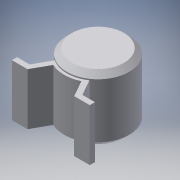
# Autodesk Inventor part: Motor
Saved by Autodesk Inventor 2019 (Build 230136000, 136)
## iProperties
Created: 2017-01-18
Part Number: Motor
Document SubType Name: Modeling
Designer: Administrator
Density: 1 g/cm^3
Mass: 12.288 g
Surface Area: 37.6061 cm^2
Volume: 12.288 cm^3
Material: Generic
Appearance: Cool White
Author: Administrator
Autodesk Inventor part; units mm, degrees
ref_plane "YZ Plane" through (0, 0, 0) normal (1, 0, 0) x (0, 1, 0)
ref_plane "XZ Plane" through (0, 0, 0) normal (0, 1, 0) x (-1, 0, 0)
ref_plane "XY Plane" through (0, 0, 0) normal (0, 0, 1) x (1, 0, 0)
sketch "Sketch1" plane through (0, 0, 0) normal (0, 0, 1) x (1, 0, 0)
  line L0 (0, 0) -> (0, -18.18) construction
  line L1 (0, -18.18) -> (-15, -18.18) construction
  line L2 (-15, -18.18) -> (-15, -16.18)
  line L3 (-15, -16.18) -> (-9, -16.18) construction
  line L4 (-9, -16.18) -> (0, 0) construction
  line L5 (-10.1443, -16.18) -> (-6.6868, -9.9643)
  line L6 (-5.4267, -11.8132) -> (-8.9682, -18.18)
  line L7 (-15, -16.18) -> (-10.1443, -16.18)
  line L8 (-15, -18.18) -> (-8.9682, -18.18)
  line L9 (15, -18.18) -> (15, -16.18)
  line L10 (15, -16.18) -> (9, -16.18) construction
  line L11 (10.1443, -16.18) -> (6.6868, -9.9643)
  line L12 (5.4267, -11.8132) -> (8.9682, -18.18)
  line L13 (15, -16.18) -> (10.1443, -16.18)
  line L14 (15, -18.18) -> (8.9682, -18.18)
  arc A0 (-5.4267, -11.8132) -> (5.4267, -11.8132) centre (0, 0) ccw
  arc A1 (6.6868, -9.9643) -> (-6.6868, -9.9643) centre (0, 0) ccw
  dimension "d1" = 15
  dimension "d2" = 18.18
  dimension "d3" = 2
  dimension "d4" = 6
  dimension "d5" = 1
  dimension "d6" = 2
  dimension "d9" = 12
  dimension "d10" = 13
  constraints: 30 end point, 7 symmetric about line, 4 parallel, 4 point on circle, 3 point on line, 2 centre point, 2 collinear, 1 perpendicular, 1 vertical, 1 other
  measures "d1" distance of L0.end L1.end
  measures "d2" distance from line of L0.start L1
  measures "d3" distance between parallel lines of L3 L1
  measures "d4" distance from line of L3.end L2
  measures "d5" distance between parallel lines of L5 L4
  measures "d6" distance between parallel lines of L5 L6
  measures "d9" radius of A1
  measures "d10" radius of A0
extrude "Extrusion1" add sketch "Sketch1" along normal mid plane 20
sketch "Sketch2" plane through (0, 0, 0) normal (0, 0, 1) x (1, 0, 0)
  arc A0 (6.6868, -9.9643) -> (-6.6868, -9.9643) centre (0, 0) ccw projected
  circle A1 centre (0, 0) radius 12
  constraints: 1 centre point, 1 coincident, 1 concentric
extrude "Extrusion2" add sketch "Sketch2" along normal mid plane 25
chamfer "Chamfer1" distance 2 angle 45 2 edges at (-12, 0, 12.5) (-12, 0, -12.5)
body "Solid1"
